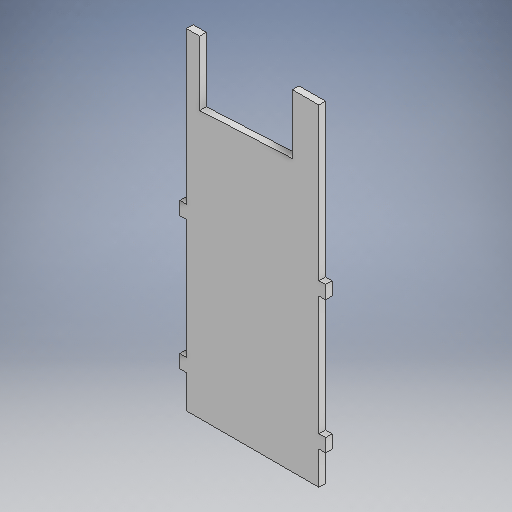
# Autodesk Inventor part: face
Saved by Autodesk Inventor 2025.3 (Build 293356000, 356)
## iProperties
Created: 2026-04-15
Part Number: face
Material: Generic
Document SubType Name: Modeling
Designer: user
Density: 1 g/cm^3
Appearance: Default
Author: user
Autodesk Inventor part; units mm, degrees
ref_plane "YZ Plane" through (0, 0, 0) normal (1, 0, 0) x (0, 1, 0)
ref_plane "XZ Plane" through (0, 0, 0) normal (0, 1, 0) x (-1, 0, 0)
ref_plane "XY Plane" through (0, 0, 0) normal (0, 0, 1) x (1, 0, 0)
sketch "Sketch1" plane through (0, 0, 0) normal (0, 0, 1) x (1, 0, 0)
  line L0 (49.4899, 15.1346) -> (44.4899, 15.1346)
  line L1 (44.4899, 15.1346) -> (44.4899, 130.0346)
  line L2 (44.4899, 130.0346) -> (24.4899, 130.0346)
  line L3 (44.4899, -119.9654) -> (49.4899, -119.9654) construction
  line L4 (44.4899, 5.1346) -> (49.4899, 5.1346)
  line L5 (-55.5101, -119.9654) -> (44.4899, -119.9654)
  line L6 (-55.5101, -119.9654) -> (-55.5101, -94.9654)
  line L7 (-55.5101, -119.9654) -> (-65.5101, -119.9654) construction
  line L8 (-55.5101, -94.9654) -> (-60.5101, -94.9654)
  line L9 (-60.5101, -94.9654) -> (-60.5101, -84.9654)
  line L10 (-60.5101, -84.9654) -> (-55.5101, -84.9654)
  line L11 (-55.5101, -84.9654) -> (-55.5101, 5.1346)
  line L12 (-55.5101, 5.1346) -> (-60.5101, 5.1346)
  line L13 (24.4899, 130.0346) -> (24.4899, 85.0346)
  line L14 (24.4899, 85.0346) -> (-45.5101, 81.3661)
  line L15 (-45.5101, 130.0346) -> (-45.5101, 81.3661)
  line L16 (-55.5101, 130.0346) -> (-45.5101, 130.0346)
  line L17 (-60.5101, 15.1346) -> (-55.5101, 15.1346)
  line L18 (-60.5101, 15.1346) -> (-55.5101, 15.1346)
  line L19 (-60.5101, 5.1346) -> (-60.5101, 15.1346)
  line L20 (-60.5101, 5.1346) -> (-60.5101, 15.1346)
  line L21 (-55.5101, 5.1346) -> (-60.5101, 5.1346)
  line L22 (49.4899, -94.9654) -> (49.4899, -84.9654)
  line L23 (44.4899, -94.9654) -> (49.4899, -94.9654)
  line L24 (44.4899, -84.9654) -> (49.4899, -84.9654)
  line L25 (49.4899, 15.1346) -> (49.4899, 5.1346)
  line L26 (-55.5101, 130.0346) -> (-55.5101, 15.1346)
  line L27 (44.4899, -119.9654) -> (44.4899, -94.9654)
  line L28 (44.4899, -84.9654) -> (44.4899, 5.1346)
  line L29 (44.4899, -16.7997) -> (64.4899, -16.7997) construction
  point P0 (0, 0)
  point P1 (-7.6774, -16.7997)
  point P2 (34.4899, 130.0346)
  dimension "d0" = 100
  dimension "d1" = 20
  dimension "d2" = 45
  dimension "d3" = 93
  dimension "d4" = 10
  dimension "d5" = 10
  dimension "d6" = 10
  dimension "d7" = 10
  dimension "d8" = 5
  dimension "d9" = 5
  dimension "d10" = 5
  dimension "d11" = 48.6685
  dimension "d12" = 250
  dimension "d13" = 47.8327
  dimension "d14" = 114.9
  dimension "d15" = 114.9
  dimension "d16" = 20
  constraints: 60 end point, 7 horizontal, 6 vertical, 3 perpendicular, 1 midpoint, 1 parallel, 1 point on line
  measures "d0" distance of L5.start L5.end
  measures "d1" distance of L1.end L2.end
  measures "d2" distance of L2.end L13.end
  measures "d3" angle of L13 L14
  measures "d4" distance of L26.start L15.start
  measures "d5" distance of L5.start L7.end
  measures "d6" distance of L8.end L10.start
  measures "d7" distance of L19.start L19.end
  measures "d8" distance of L19.end L17.end
  measures "d9" distance of L4.start L25.end
  measures "d10" distance of L10.start L11.start
  measures "d11" distance of L15.start L15.end
  measures "d12" distance from line of L5 point (34.49, 130.035)
  measures "d13" distance from line of L11 point (-7.677, -16.8)
  measures "d14" distance of L1.start L1.end
  measures "d15" distance of L26.start L17.end
  measures "d16" distance of L29.start L29.end
extrude "Extrusion1" add sketch "Sketch1" along normal blind 5
body "Solid1"
